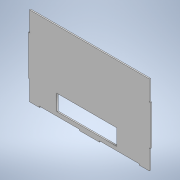
# Autodesk Inventor part: Base lateral
Saved by Autodesk Inventor 2020 (Build 240168000, 168)
## iProperties
Created: 2020-03-15
Part Number: Base lateral
Material: Genérico
Document SubType Name: Modeling
Designer: JRoCC97
Density: 1 g/cm^3
Appearance: Valor por defecto
Author: JRoCC97
Autodesk Inventor part; units mm, degrees
ref_plane "YZ Plane" through (0, 0, 0) normal (1, 0, 0) x (0, 1, 0)
ref_plane "XZ Plane" through (0, 0, 0) normal (0, 1, 0) x (-1, 0, 0)
ref_plane "XY Plane" through (0, 0, 0) normal (0, 0, 1) x (1, 0, 0)
sketch "Boceto1" plane through (0, 0, 0) normal (0, 0, 1) x (1, 0, 0)
  line L0 (0, 200) -> (300, 200)
  line L1 (25, 0) -> (25, 3)
  line L2 (25, 3) -> (125, 3)
  line L3 (125, 3) -> (125, 0)
  line L4 (175, 0) -> (175, 3)
  line L5 (175, 3) -> (275, 3)
  line L6 (275, 3) -> (275, 0)
  line L7 (25, 0) -> (0, 0)
  line L8 (300, 0) -> (275, 0)
  line L9 (175, 0) -> (125, 0)
  line L10 (0, 150) -> (-3, 150)
  line L11 (-3, 150) -> (-3, 50)
  line L12 (-3, 50) -> (0, 50)
  line L13 (0, 0) -> (0, 50)
  line L14 (0, 150) -> (0, 200)
  line L15 (300, 150) -> (303, 150)
  line L16 (303, 150) -> (303, 50)
  line L17 (303, 50) -> (300, 50)
  line L18 (300, 200) -> (300, 150)
  line L19 (300, 50) -> (300, 0)
  dimension "d4" = 100
  dimension "d6" = 100
  dimension "d10" = 50
  dimension "d13" = 3
  dimension "d14" = 200
  dimension "d15" = 3
  dimension "d16" = 100
  dimension "d17" = 50
  dimension "d21" = 300
  constraints: 40 end point, 16 perpendicular, 7 parallel, 6 collinear, 3 horizontal, 2 equal length, 2 vertical, 1 coincident
  measures "d4" distance of L1.end L2.end
  measures "d6" distance of L4.end L5.end
  measures "d10" distance between parallel lines of L4 L3
  measures "d13" distance between parallel lines of L7 L2
  measures "d14" distance between parallel lines of L0 L8
  measures "d15" distance of L10.start L10.end
  measures "d16" distance of L10.end L11.end
  measures "d17" distance between parallel lines of L0 L10
  measures "d21" distance between parallel lines of L14 L18
extrude "Extrusión1" add sketch "Boceto1" along normal blind 3
sketch "Boceto2" plane through (0, 0, 3) normal (0, 0, 1) x (1, 0, 0)
  line L0 (68.5, 53) -> (218.5, 53)
  line L1 (218.5, 53) -> (218.5, 13)
  line L2 (218.5, 13) -> (68.5, 13)
  line L3 (68.5, 13) -> (68.5, 53)
  line L4 (0, 50) -> (0, 0) projected
  line L5 (25, 3) -> (125, 3) projected
  dimension "d22" = 40
  dimension "d23" = 150
  dimension "d26" = 68.5
  dimension "d27" = 10
  constraints: 8 end point, 2 parallel, 1 horizontal, 1 perpendicular
  measures "d22" distance between parallel lines of L2 L0
  measures "d23" distance between parallel lines of L1 L3
  measures "d26" distance between parallel lines of L4 L3
  measures "d27" distance between parallel lines of L5 L2
extrude "Extrusión2" cut sketch "Boceto2" against normal blind 3
